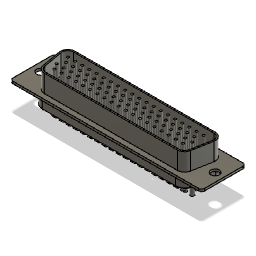
39_2part (Autodesk Fusion 360 design; units mm, degrees)
Autodesk Fusion 360 part; units mm, degrees
sketch "Sketch1" plane through (0, 0, 0) normal (0, 1, 0) x (1, 0, 0)
  line L0 (-32.5, 7.75) -> (32.5, 7.75)
  line L1 (33.5, 6.75) -> (33.5, -6.75)
  line L2 (32.5, -7.75) -> (-32.5, -7.75)
  line L3 (-33.5, -6.75) -> (-33.5, 6.75)
  arc A0 (33.5, 6.75) -> (32.5, 7.75) centre (32.5, 6.75) ccw
  arc A1 (32.5, -7.75) -> (33.5, -6.75) centre (32.5, -6.75) ccw
  arc A2 (-33.5, -6.75) -> (-32.5, -7.75) centre (-32.5, -6.75) ccw
  arc A3 (-32.5, 7.75) -> (-33.5, 6.75) centre (-32.5, 6.75) ccw
  line L4 (-85.3227, 0) -> (66.5098, 0) construction
  line L5 (0, 50.6733) -> (0, -34.9257) construction
  circle A4 centre (30.5, 0) radius 1.5
  circle A5 centre (-30.5, 0) radius 1.5
  line L6 (-24.6036, 5.5) -> (24.6036, 5.5)
  line L7 (26.5713, 3.1422) -> (25.2986, -3.8578)
  line L8 (23.3308, -5.5) -> (-23.3308, -5.5)
  line L9 (-25.2986, -3.8578) -> (-26.5713, 3.1422)
  arc A6 (26.5713, 3.1422) -> (24.6036, 5.5) centre (24.6036, 3.5) ccw
  arc A7 (23.3308, -5.5) -> (25.2986, -3.8578) centre (23.3308, -3.5) ccw
  arc A8 (-25.2986, -3.8578) -> (-23.3308, -5.5) centre (-23.3308, -3.5) ccw
  arc A9 (-24.6036, 5.5) -> (-26.5713, 3.1422) centre (-24.6036, 3.5) ccw
  circle A10 centre (23.4963, 3) radius 0.4
  circle A11 centre (20.9963, 3) radius 0.4
  circle A12 centre (18.4963, 3) radius 0.4
  circle A13 centre (15.9963, 3) radius 0.4
  circle A14 centre (13.4963, 3) radius 0.4
  circle A15 centre (10.9963, 3) radius 0.4
  circle A16 centre (8.4963, 3) radius 0.4
  circle A17 centre (5.9963, 3) radius 0.4
  circle A18 centre (3.4963, 3) radius 0.4
  circle A19 centre (0.9963, 3) radius 0.4
  circle A20 centre (-1.5037, 3) radius 0.4
  circle A21 centre (-4.0037, 3) radius 0.4
  circle A22 centre (-6.5037, 3) radius 0.4
  circle A23 centre (-9.0037, 3) radius 0.4
  circle A24 centre (-11.5037, 3) radius 0.4
  circle A25 centre (-14.0037, 3) radius 0.4
  circle A26 centre (-16.5037, 3) radius 0.4
  circle A27 centre (-19.0037, 3) radius 0.4
  circle A28 centre (-21.5037, 3) radius 0.4
  circle A29 centre (-24.0037, 3) radius 0.4
  circle A30 centre (23.4963, -1) radius 0.4
  circle A31 centre (20.9963, -1) radius 0.4
  circle A32 centre (18.4963, -1) radius 0.4
  circle A33 centre (15.9963, -1) radius 0.4
  circle A34 centre (13.4963, -1) radius 0.4
  circle A35 centre (10.9963, -1) radius 0.4
  circle A36 centre (8.4963, -1) radius 0.4
  circle A37 centre (5.9963, -1) radius 0.4
  circle A38 centre (3.4963, -1) radius 0.4
  circle A39 centre (0.9963, -1) radius 0.4
  circle A40 centre (-1.5037, -1) radius 0.4
  circle A41 centre (-4.0037, -1) radius 0.4
  circle A42 centre (-6.5037, -1) radius 0.4
  circle A43 centre (-9.0037, -1) radius 0.4
  circle A44 centre (-11.5037, -1) radius 0.4
  circle A45 centre (-14.0037, -1) radius 0.4
  circle A46 centre (-16.5037, -1) radius 0.4
  circle A47 centre (-19.0037, -1) radius 0.4
  circle A48 centre (-21.5037, -1) radius 0.4
  circle A49 centre (-24.0037, -1) radius 0.4
  line L10 (20.9963, 3) -> (23.4963, -1) construction
  line L11 (23.4963, 3) -> (20.9963, -1) construction
  circle A50 centre (22.2463, 1) radius 0.4
  circle A51 centre (19.7463, 1) radius 0.4
  circle A52 centre (17.2463, 1) radius 0.4
  circle A53 centre (14.7463, 1) radius 0.4
  circle A54 centre (12.2463, 1) radius 0.4
  circle A55 centre (9.7463, 1) radius 0.4
  circle A56 centre (7.2463, 1) radius 0.4
  circle A57 centre (4.7463, 1) radius 0.4
  circle A58 centre (2.2463, 1) radius 0.4
  circle A59 centre (-0.2537, 1) radius 0.4
  circle A60 centre (-2.7537, 1) radius 0.4
  circle A61 centre (-5.2537, 1) radius 0.4
  circle A62 centre (-7.7537, 1) radius 0.4
  circle A63 centre (-10.2537, 1) radius 0.4
  circle A64 centre (-12.7537, 1) radius 0.4
  circle A65 centre (-15.2537, 1) radius 0.4
  circle A66 centre (-17.7537, 1) radius 0.4
  circle A67 centre (-20.2537, 1) radius 0.4
  circle A68 centre (-22.7537, 1) radius 0.4
  circle A69 centre (22.2463, -3) radius 0.4
  circle A70 centre (19.7463, -3) radius 0.4
  circle A71 centre (17.2463, -3) radius 0.4
  circle A72 centre (14.7463, -3) radius 0.4
  circle A73 centre (12.2463, -3) radius 0.4
  circle A74 centre (9.7463, -3) radius 0.4
  circle A75 centre (7.2463, -3) radius 0.4
  circle A76 centre (4.7463, -3) radius 0.4
  circle A77 centre (2.2463, -3) radius 0.4
  circle A78 centre (-0.2537, -3) radius 0.4
  circle A79 centre (-2.7537, -3) radius 0.4
  circle A80 centre (-5.2537, -3) radius 0.4
  circle A81 centre (-7.7537, -3) radius 0.4
  circle A82 centre (-10.2537, -3) radius 0.4
  circle A83 centre (-12.7537, -3) radius 0.4
  circle A84 centre (-15.2537, -3) radius 0.4
  circle A85 centre (-17.7537, -3) radius 0.4
  circle A86 centre (-20.2537, -3) radius 0.4
  circle A87 centre (-22.7537, -3) radius 0.4
  arc A88 (-25.7905, -3.9472) -> (-23.3308, -6) centre (-23.3308, -3.5) ccw
  line L12 (23.3308, -6) -> (-23.3308, -6)
  arc A89 (23.3308, -6) -> (25.7905, -3.9472) centre (23.3308, -3.5) ccw
  line L13 (27.0632, 3.0528) -> (25.7905, -3.9472)
  arc A90 (27.0632, 3.0528) -> (24.6036, 6) centre (24.6036, 3.5) ccw
  line L14 (-24.6036, 6) -> (24.6036, 6)
  arc A91 (-24.6036, 6) -> (-27.0632, 3.0528) centre (-24.6036, 3.5) ccw
  line L15 (-25.7905, -3.9472) -> (-27.0632, 3.0528)
  arc A92 (-26.4792, -4.0724) -> (-23.3308, -6.7) centre (-23.3308, -3.5) ccw
  line L16 (23.3308, -6.7) -> (-23.3308, -6.7)
  arc A93 (23.3308, -6.7) -> (26.4792, -4.0724) centre (23.3308, -3.5) ccw
  line L17 (27.752, 2.9276) -> (26.4792, -4.0724)
  arc A94 (27.752, 2.9276) -> (24.6036, 6.7) centre (24.6036, 3.5) ccw
  line L18 (-24.6036, 6.7) -> (24.6036, 6.7)
  arc A95 (-24.6036, 6.7) -> (-27.752, 2.9276) centre (-24.6036, 3.5) ccw
  line L19 (-26.4792, -4.0724) -> (-27.752, 2.9276)
  point P0 (-33.5, 7.75)
  point P1 (33.5, 7.75)
  point P2 (-33.5, -7.75)
  point P3 (-27, 5.5)
  point P4 (27, 5.5)
  point P5 (25, -5.5)
  point P6 (-25, -5.5)
  dimension "d1" = 67
  dimension "d2" = 15.5
  dimension "d3" = 1
  dimension "d4" = 1
  dimension "d5" = 1
  dimension "d6" = 1
  dimension "d7" = 3
  dimension "d8" = 3
  dimension "d9" = 11
  dimension "d10" = 54
  dimension "d11" = 50
  dimension "d12" = 2
  dimension "d13" = 2
  dimension "d14" = 2
  dimension "d15" = 2
  dimension "d16" = 0.8
  dimension "d17" = 2.5
  dimension "d18" = 3
  dimension "d21" = -2.5
  dimension "d22" = -4
  dimension "d25" = -2.5
  dimension "d26" = -4
  dimension "d27" = -0.5
  dimension "d32" = -1.2
  constraint horizontal L0
  constraint vertical L1
  constraint horizontal L2
  constraint vertical L3
  constraint coincident P1 L0
  constraint coincident P1 L1
  constraint tangent L0 A0
  constraint tangent L1 A0
  constraint tangent L1 A1
  constraint tangent L2 A1
  constraint coincident P2 L2
  constraint coincident P2 L3
  constraint tangent L2 A2
  constraint tangent L3 A2
  constraint coincident P0 L3
  constraint coincident P0 L0
  constraint tangent L3 A3
  constraint tangent L0 A3
  constraint horizontal L4
  constraint coincident origin L4
  constraint vertical L5
  constraint coincident origin L5
  constraint symmetric L1 L3 L5
  constraint symmetric L0 L2 L4
  constraint coincident L4 A4.centre
  constraint symmetric L5 A4 A5
  constraint perpendicular L5 L6
  constraint perpendicular L5 L8
  constraint symmetric L5 L7 L9
  constraint coincident P4 L6
  constraint coincident P4 L7
  constraint tangent L6 A6
  constraint tangent L7 A6
  constraint coincident P5 L7
  constraint coincident P5 L8
  constraint tangent L7 A7
  constraint tangent L8 A7
  constraint coincident P6 L8
  constraint coincident P6 L9
  constraint tangent L8 A8
  constraint tangent L9 A8
  constraint coincident P3 L9
  constraint coincident P3 L6
  constraint tangent L9 A9
  constraint tangent L6 A9
  constraint coincident A11.centre L10.start
  constraint coincident A30.centre L10.end
  constraint coincident A10.centre L11.start
  constraint coincident A31.centre L11.end
  constraint midpoint L11 A50.centre
  constraint equal A10 A50
  measures "d1" distance of P0 P1
  measures "d2" distance of P0 P2
  measures "d3" radius of A0
  measures "d4" radius of A1
  measures "d5" radius of A2
  measures "d6" radius of A3
  measures "d7" diameter of A4
  measures "d8" distance of L1 A4.centre
  measures "d9" distance of L6 L8
  measures "d10" distance of P3 P4
  measures "d11" distance of P5 P6
  measures "d12" radius of A6
  measures "d13" radius of A7
  measures "d14" radius of A8
  measures "d15" radius of A9
  measures "d16" diameter of A10
  measures "d17" distance of L6 A10.centre
  measures "d18" distance of L7 A10.centre
extrude "Extrude1" add sketch "Sketch1" along normal blind 0.8 contours L0 L1 L2 L3 A0 A1 A2 A3 | A92 L16 A93 L17 A94 L18 A95 L19 makes body 1
extrude "Extrude2" add sketch "Sketch1" along normal blind 7 separate body contours A10 | A11 | A12 | A13 | A14 | A15 | A16 | A17 | A18 | A19 | A20 | A21 | A22 | A23 | A24 | A25 | A26 | A27 | A28 | A29 | A30 | A31 | A32 | A33 | A34 | A35 | A36 | A37 | A38 | A39 | A40 | A41 | A42 | A43 | A44 | A45 | A46 | A47 | A48 | A49 | A50 | A51 | A52 | A53 | A54 | A55 | A56 | A57 | A58 | A59 | A60 | A61 | A62 | A63 | A64 | A65 | A66 | A67 | A68 | A69 | A70 | A71 | A72 | A73 | A74 | A75 | A76 | A77 | A78 | A79 | A80 | A81 | A82 | A83 | A84 | A85 | A86 | A87 | A88 L12 A89 L13 A90 L14 A91 L15 makes body 2 at (23.4863, 4.6667, 0.6001) makes body 3 at (20.9863, 4.6667, -3.3999) makes body 4 at (15.1443, 4.6667, 3.0398) makes body 5 at (16.1237, 4.6667, -3.3792) makes body 6 at (10.1443, 4.6667, 3.0398) makes body 7 at (11.3943, 4.6667, -2.9602) makes body 8 at (5.1443, 4.6667, 3.0398) makes body 9 at (6.3943, 4.6667, -2.9602) makes body 10 at (0.1443, 4.6667, 3.0398) makes body 11 at (1.3943, 4.6667, -2.9602) makes body 12 at (-4.8557, 4.6667, 3.0398) makes body 13 at (-3.6057, 4.6667, -2.9602) makes body 14 at (-9.8557, 4.6667, 3.0398) makes body 15 at (-8.6057, 4.6667, -2.9602) makes body 16 at (-8.2012, 4.6667, -6) makes body 17 at (-11.1057, 4.6667, -2.9602) makes body 18 at (-17.7637, 4.6667, 2.6001) makes body 19 at (-20.2637, 4.6667, 2.6001) makes body 20 at (-22.7637, 4.6667, 2.6001) makes body 21 at (-24.0137, 4.6667, -3.3999) makes body 22 at (-24.0137, 4.6667, 0.6001) makes body 23 at (-19.0137, 4.6667, -3.3999) makes body 24 at (-16.5137, 4.6667, -3.3999) makes body 25 at (-13.6057, 4.6667, -2.9602) makes body 26 at (-14.8557, 4.6667, 3.0398) makes body 27 at (-9.8557, 4.6667, -0.9602) makes body 28 at (-8.6057, 4.6667, 1.0398) makes body 29 at (-4.8557, 4.6667, -0.9602) makes body 30 at (-3.6057, 4.6667, 1.0398) makes body 31 at (0.1443, 4.6667, -0.9602) makes body 32 at (1.3943, 4.6667, 1.0398) makes body 33 at (5.1443, 4.6667, -0.9602) makes body 34 at (6.3943, 4.6667, 1.0398) makes body 35 at (10.1443, 4.6667, -0.9602) makes body 36 at (11.3943, 4.6667, 1.0398) makes body 37 at (15.1443, 4.6667, -0.9602) makes body 38 at (16.1046, 2.3333, 1.385) makes body 39 at (19.7363, 4.6667, -1.3999) makes body 40 at (20.9863, 4.6667, 0.6001) makes body 41 at (22.2363, 4.6667, 2.6001) makes body 42 at (23.4863, 4.6667, -3.3999) makes body 43 at (17.2363, 4.6667, 2.6001) makes body 44 at (18.4863, 4.6667, -3.3999) makes body 45 at (12.6443, 4.6667, 3.0398) makes body 46 at (13.8943, 4.6667, -2.9602) makes body 47 at (7.6443, 4.6667, 3.0398) makes body 48 at (8.8943, 4.6667, -2.9602) makes body 49 at (2.6443, 4.6667, 3.0398) makes body 50 at (3.8943, 4.6667, -2.9602) makes body 51 at (-2.3557, 4.6667, 3.0398) makes body 52 at (-1.1057, 4.6667, -2.9602) makes body 53 at (-7.3557, 4.6667, 3.0398) makes body 54 at (-6.1057, 4.6667, -2.9602) makes body 55 at (-12.3557, 4.6667, 3.0398) makes body 56 at (-12.3557, 4.6667, -0.9602) makes body 57 at (-16.5137, 4.6667, 0.6001) makes body 58 at (-19.0137, 4.6667, 0.6001) makes body 59 at (-21.5137, 4.6667, 0.6001) makes body 60 at (-21.5137, 4.6667, -3.3999) makes body 61 at (-22.7637, 4.6667, -1.3999) makes body 62 at (-20.2637, 4.6667, -1.3999) makes body 63 at (-17.7637, 4.6667, -1.3999) makes body 64 at (-14.8557, 4.6667, -0.9602) makes body 65 at (-13.6057, 4.6667, 1.0398) makes body 66 at (-11.1057, 4.6667, 1.0398) makes body 67 at (-7.3557, 4.6667, -0.9602) makes body 68 at (-6.1057, 4.6667, 1.0398) makes body 69 at (-2.3557, 4.6667, -0.9602) makes body 70 at (-1.1057, 4.6667, 1.0398) makes body 71 at (2.6443, 4.6667, -0.9602) makes body 72 at (3.8943, 4.6667, 1.0398) makes body 73 at (7.6443, 4.6667, -0.9602) makes body 74 at (8.8943, 4.6667, 1.0398) makes body 75 at (12.6443, 4.6667, -0.9602) makes body 76 at (13.8943, 4.6667, 1.0398) makes body 77 at (17.2363, 4.6667, -1.3999) makes body 78 at (18.4863, 4.6667, 0.6001) makes body 79 at (22.2363, 4.6667, -1.3999) makes body 80 at (19.7363, 4.6667, 2.6001)
extrude "Extrude3" add sketch "Sketch1" against normal blind 4 contours L6 L7 L8 L9 A6 A7 A8 A9 | A88 L12 A89 L13 A90 L14 A91 L15 | A92 L16 A93 L17 A94 L18 A95 L19 bodies 1 2
fillet "Fillet1" radius 0.5 8 edges at (27.0604, -4, -5.5504) (27.1156, -4, 0.5724) (25.3812, -4, 5.9568) (0, -4, 6.7) (-25.3812, -4, 5.9568) (-27.1156, -4, 0.5724) (-27.0604, -4, -5.5504) (0, -4, -6.7) on bodies 1
extrude "Extrude4" add sketch "Sketch1" against normal blind 7 contours A10 | A11 | A12 | A13 | A14 | A15 | A16 | A17 | A18 | A19 | A20 | A21 | A22 | A23 | A24 | A25 | A26 | A27 | A28 | A29 | A69 | A70 | A71 | A72 | A73 | A74 | A75 | A76 | A77 | A78 | A79 | A80 | A81 | A82 | A83 | A84 | A85 | A86 | A87 bodies 1
extrude "Extrude5" add sketch "Sketch1" against normal blind 9 contours A30 | A31 | A32 | A33 | A34 | A35 | A36 | A37 | A38 | A39 | A40 | A41 | A42 | A43 | A44 | A45 | A46 | A47 | A48 | A49 | A50 | A51 | A52 | A53 | A54 | A55 | A56 | A57 | A58 | A59 | A60 | A61 | A62 | A63 | A64 | A65 | A66 | A67 | A68 bodies 1
move_face "OffsetFaces1" offset 0.3 78 faces at (-23.9938, -5.6667, 0.6001) (-22.7438, -5.6667, -1.3999) (-23.9938, -6, -3.3999) (-22.7438, -6, 2.6001) (-20.2438, -6, 2.6001) (-21.4938, -5.6667, 0.6001) (-20.2438, -5.6667, -1.3999) (-21.4938, -6, -3.3999) (-18.9938, -6, -3.3999) (-17.7438, -5.6667, -1.3999) (-16.4938, -5.6667, 0.6001) (-17.7438, -6, 2.6001) (-14.8557, -5, 3.0398) (-13.6057, -5.6667, 1.0398) (-14.8557, -5.6667, -0.9602) (-16.4938, -6, -3.3999) (-13.6057, -5, -2.9602) (-12.3557, -5.6667, -0.9602) (-18.9938, -5.6667, 0.6001) (-12.3557, -5, 3.0398) (-11.1057, -5.6667, 1.0398) (-9.8557, -5.6667, -0.9602) (-11.1057, -5, -2.9602) (-8.6057, -5, -2.9602) (-6.1057, -5, -2.9602) (-3.6057, -5, -2.9602) (-1.1057, -5, -2.9602) (1.3943, -5, -2.9602) (3.8943, -5, -2.9602) (6.3943, -5, -2.9602) (8.8943, -5, -2.9602) (11.3943, -5, -2.9602) (-7.3557, -5.6667, -0.9602) (-4.8557, -5.6667, -0.9602) (7.6443, -5.6667, -0.9602) (10.1443, -5.6667, -0.9602) (12.6443, -5.6667, -0.9602) (15.1443, -5.6667, -0.9602) (17.2562, -5.6667, -1.3999) (-2.3557, -5.6667, -0.9602) (0.1443, -5.6667, -0.9602) (2.6443, -5.6667, -0.9602) (5.1443, -5.6667, -0.9602) (-8.6057, -5.6667, 1.0398) (-9.8557, -5, 3.0398) (-7.3557, -5, 3.0398) (-6.1057, -5.6667, 1.0398) (-4.8557, -5, 3.0398) (-3.6057, -5.6667, 1.0398) (-2.3557, -5, 3.0398) (0.1443, -5, 3.0398) (1.3943, -5.6667, 1.0398) (2.6443, -5, 3.0398) (3.8943, -5.6667, 1.0398) (10.1443, -5, 3.0398) (12.6443, -5, 3.0398) (13.8943, -5.6667, 1.0398) (15.1443, -5, 3.0398) (16.1046, -7.3333, 1.385) (-1.1057, -5.6667, 1.0398) (7.6443, -5, 3.0398) (6.3943, -5.6667, 1.0398) (8.8943, -5.6667, 1.0398) (11.3943, -5.6667, 1.0398) (17.2562, -6, 2.6001) (19.7562, -6, 2.6001) (22.2562, -6, 2.6001) (23.5062, -5.6667, 0.6001) (21.0062, -5.6667, 0.6001) (18.5062, -5.6667, 0.6001) (19.7562, -5.6667, -1.3999) (22.2562, -5.6667, -1.3999) (18.5062, -6, -3.3999) (16.1237, -5, -3.3792) (13.8943, -5, -2.9602) (5.1443, -5, 3.0398) (21.0062, -6, -3.3999) (23.5062, -6, -3.3999) on bodies 1
extrude "Extrude6" cut sketch "Sketch1" against normal blind 9 contours A10 | A11 | A12 | A13 | A14 | A15 | A16 | A17 | A18 | A19 | A20 | A21 | A22 | A23 | A24 | A25 | A26 | A27 | A28 | A29 | A30 | A31 | A32 | A33 | A34 | A35 | A36 | A37 | A38 | A39 | A40 | A41 | A42 | A43 | A44 | A45 | A46 | A47 | A48 | A49 | A50 | A51 | A52 | A53 | A54 | A55 | A56 | A57 | A58 | A59 | A60 | A61 | A62 | A63 | A64 | A65 | A66 | A67 | A68 | A69 | A70 | A71 | A72 | A73 | A74 | A75 | A76 | A77 | A78 | A79 | A80 | A81 | A82 | A83 | A84 | A85 | A86 | A87 bodies 1
